Autodesk Fusion 360 part; units mm, degrees
(part 5 of 6)
ref_plane "WorkPlane4" through (0, 0, 43.2) normal (0, 0, 1) x (1, 0, 0) in component "USB — removable rear housing clamp"
sketch "USB clamp upper strap extension sketch" plane through (0, 0, 43.2) normal (0, 0, 1) x (1, 0, 0) in component "USB — removable rear housing clamp"
  line L0 (65.7, 19.7) -> (72.4, 19.7)
  line L1 (72.4, 19.7) -> (72.4, 25)
  line L2 (72.4, 25) -> (65.7, 25)
  line L3 (65.7, 25) -> (65.7, 19.7)
  dimension "d2143" = 65.7
  dimension "d2144" = 19.7
  dimension "d2145" = 6.7
  dimension "d2146" = 5.3
  constraint horizontal L0
  constraint vertical L1
  constraint horizontal L2
  constraint vertical L3
  measures "d2143" horizontal distance of origin L0.start
  measures "d2144" vertical distance of origin L0.start
  measures "d2145" horizontal distance of L0.start L0.end
  measures "d2146" vertical distance of L0.end L1.end
extrude "USB clamp upper strap extension" add sketch "USB clamp upper strap extension sketch" along normal blind 2 bodies 61 in component "USB — removable rear housing clamp"
ref_plane "WorkPlane5" through (0, 0, 35) normal (0, 0, 1) x (1, 0, 0) in component "USB — removable rear housing clamp"
sketch "USB clamp upper inward-stop stalk sketch" plane through (0, 0, 35) normal (0, 0, 1) x (1, 0, 0) in component "USB — removable rear housing clamp"
  line L0 (68.4, 23) -> (70.4, 23)
  line L1 (70.4, 23) -> (70.4, 25)
  line L2 (70.4, 25) -> (68.4, 25)
  line L3 (68.4, 25) -> (68.4, 23)
  dimension "d2151" = 68.4
  dimension "d2152" = 23
  dimension "d2153" = 2
  dimension "d2154" = 2
  constraint horizontal L0
  constraint vertical L1
  constraint horizontal L2
  constraint vertical L3
  measures "d2151" horizontal distance of origin L0.start
  measures "d2152" vertical distance of origin L0.start
  measures "d2153" horizontal distance of L0.start L0.end
  measures "d2154" vertical distance of L0.end L1.end
extrude "USB clamp upper inward-stop stalk" add sketch "USB clamp upper inward-stop stalk sketch" along normal blind 8.3 bodies 61 in component "USB — removable rear housing clamp"
ref_plane "WorkPlane6" through (0, 0, 34.9) normal (0, 0, 1) x (1, 0, 0) in component "USB — removable rear housing clamp"
sketch "Clear lower rear-cover boss from USB clamp sketch" plane through (0, 0, 34.9) normal (0, 0, 1) x (1, 0, 0) in component "USB — removable rear housing clamp"
  line L0 (65.6, 8.4) -> (72.5, 8.4)
  line L1 (72.5, 8.4) -> (72.5, 12)
  line L2 (72.5, 12) -> (65.6, 12)
  line L3 (65.6, 12) -> (65.6, 8.4)
  dimension "d2159" = 65.6
  dimension "d2160" = 8.4
  dimension "d2161" = 6.9
  dimension "d2162" = 3.6
  constraint horizontal L0
  constraint vertical L1
  constraint horizontal L2
  constraint vertical L3
  measures "d2159" horizontal distance of origin L0.start
  measures "d2160" vertical distance of origin L0.start
  measures "d2161" horizontal distance of L0.start L0.end
  measures "d2162" vertical distance of L0.end L1.end
extrude "Clear lower rear-cover boss from USB clamp" cut sketch "Clear lower rear-cover boss from USB clamp sketch" along normal blind 10.4 bodies 61 in component "USB — removable rear housing clamp"
ref_plane "WorkPlane1" through (0, 0, 21.25) normal (0, 0, 1) x (1, 0, 0)
sketch "USB parametric mounting point 2" plane through (0, 0, 21.25) normal (0, 0, 1) x (1, 0, 0)
  circle A0 centre (74.9, 8.25) radius 0.1
  dimension "d2175" = 74.9
  dimension "d2176" = 8.25
  dimension "d2177" = 0.1
  measures "d2175" horizontal distance of origin A0.centre
  measures "d2176" vertical distance of origin A0.centre
  measures "d2177" radius of A0
sketch "Negative Z orientation datum 2" plane through (0, 0, 0) normal (0, 1, 0) x (1, 0, 0)
  line L0 (0, 0) -> (0, 10)
ref_plane "WorkPlane2" through (0, 0, 30.95) normal (0, 0, 1) x (1, 0, 0)
sketch "USB parametric mounting point 6" plane through (0, 0, 30.95) normal (0, 0, 1) x (1, 0, 0)
  circle A0 centre (74.9, 23.75) radius 0.1
  dimension "d2212" = 74.9
  dimension "d2213" = 23.75
  dimension "d2214" = 0.1
  measures "d2212" horizontal distance of origin A0.centre
  measures "d2213" vertical distance of origin A0.centre
  measures "d2214" radius of A0
sketch "Negative Z orientation datum 6" plane through (0, 0, 0) normal (0, 1, 0) x (1, 0, 0)
  line L0 (0, 0) -> (0, 10)
ref_plane "WorkPlane3" through (0, 0, 21.25) normal (0, 0, 1) x (1, 0, 0)
sketch "USB parametric mounting point 7" plane through (0, 0, 21.25) normal (0, 0, 1) x (1, 0, 0)
  circle A0 centre (72.6, 8.25) radius 0.1
  dimension "d2225" = 72.6
  dimension "d2226" = 8.25
  dimension "d2227" = 0.1
  measures "d2225" horizontal distance of origin A0.centre
  measures "d2226" vertical distance of origin A0.centre
  measures "d2227" radius of A0
sketch "Negative Z orientation datum 7" plane through (0, 0, 0) normal (0, 1, 0) x (1, 0, 0)
  line L0 (0, 0) -> (0, 10)
ref_plane "WorkPlane4" through (0, 0, 30.95) normal (0, 0, 1) x (1, 0, 0)
sketch "USB parametric mounting point 8" plane through (0, 0, 30.95) normal (0, 0, 1) x (1, 0, 0)
  circle A0 centre (72.6, 23.75) radius 0.1
  dimension "d2238" = 72.6
  dimension "d2239" = 23.75
  dimension "d2240" = 0.1
  measures "d2238" horizontal distance of origin A0.centre
  measures "d2239" vertical distance of origin A0.centre
  measures "d2240" radius of A0
sketch "Negative Z orientation datum 8" plane through (0, 0, 0) normal (0, 1, 0) x (1, 0, 0)
  line L0 (0, 0) -> (0, 10)
ref_plane "WorkPlane1" through (0, 0, 16.5) normal (0, 0, 1) x (1, 0, 0) in component "Chamber / sealed L cartridge concept"
sketch "L sampling cartridge sketch" plane through (0, 0, 16.5) normal (0, 0, 1) x (1, 0, 0) in component "Chamber / sealed L cartridge concept"
  line L0 (2.9, 87) -> (72.1, 87)
  line L1 (72.1, 87) -> (72.1, 122.1)
  line L2 (72.1, 122.1) -> (2.9, 122.1)
  line L3 (2.9, 122.1) -> (2.9, 87)
  dimension "d2267" = 2.9
  dimension "d2268" = 87
  constraint horizontal L0
  constraint vertical L1
  constraint horizontal L2
  constraint vertical L3
  measures "d2267" horizontal distance of origin L0.start
  measures "d2268" vertical distance of origin L0.start
extrude "L sampling cartridge" add sketch "L sampling cartridge sketch" along normal blind 32.3 separate body makes body 85 in component "Chamber / sealed L cartridge concept"
ref_plane "WorkPlane2" through (0, 0, 16.5) normal (0, 0, 1) x (1, 0, 0) in component "Chamber / sealed L cartridge concept"
sketch "L sampling cartridge side column sketch" plane through (0, 0, 16.5) normal (0, 0, 1) x (1, 0, 0) in component "Chamber / sealed L cartridge concept"
  line L0 (45.6, 30) -> (72.1, 30)
  line L1 (72.1, 30) -> (72.1, 122.1)
  line L2 (72.1, 122.1) -> (45.6, 122.1)
  line L3 (45.6, 122.1) -> (45.6, 30)
  dimension "d2275" = 45.6
  dimension "d2276" = 30
  constraint horizontal L0
  constraint vertical L1
  constraint horizontal L2
  constraint vertical L3
  measures "d2275" horizontal distance of origin L0.start
  measures "d2276" vertical distance of origin L0.start
extrude "L sampling cartridge side column" add sketch "L sampling cartridge side column sketch" along normal blind 32.3 bodies 85 in component "Chamber / sealed L cartridge concept"
ref_plane "WorkPlane3" through (0, 0, 18.5) normal (0, 0, 1) x (1, 0, 0) in component "Chamber / sealed L cartridge concept"
sketch "Direct upper gas cavity sketch" plane through (0, 0, 18.5) normal (0, 0, 1) x (1, 0, 0) in component "Chamber / sealed L cartridge concept"
  line L0 (4.9, 89) -> (70.1, 89)
  line L1 (70.1, 89) -> (70.1, 120.1)
  line L2 (70.1, 120.1) -> (4.9, 120.1)
  line L3 (4.9, 120.1) -> (4.9, 89)
  dimension "d2283" = 4.9
  dimension "d2284" = 89
  dimension "d2285" = 65.2
  dimension "d2286" = 31.1
  constraint horizontal L0
  constraint vertical L1
  constraint horizontal L2
  constraint vertical L3
  measures "d2283" horizontal distance of origin L0.start
  measures "d2284" vertical distance of origin L0.start
  measures "d2285" horizontal distance of L0.start L0.end
  measures "d2286" vertical distance of L0.end L1.end
extrude "Direct upper gas cavity" cut sketch "Direct upper gas cavity sketch" along normal blind 56 bodies 85 in component "Chamber / sealed L cartridge concept"
ref_plane "WorkPlane4" through (0, 0, 18.5) normal (0, 0, 1) x (1, 0, 0) in component "Chamber / sealed L cartridge concept"
sketch "Direct connected side gas cavity sketch" plane through (0, 0, 18.5) normal (0, 0, 1) x (1, 0, 0) in component "Chamber / sealed L cartridge concept"
  line L0 (47.6, 32) -> (70.1, 32)
  line L1 (70.1, 32) -> (70.1, 120.1)
  line L2 (70.1, 120.1) -> (47.6, 120.1)
  line L3 (47.6, 120.1) -> (47.6, 32)
  dimension "d2291" = 47.6
  dimension "d2292" = 32
  dimension "d2293" = 22.5
  dimension "d2294" = 88.1
  constraint horizontal L0
  constraint vertical L1
  constraint horizontal L2
  constraint vertical L3
  measures "d2291" horizontal distance of origin L0.start
  measures "d2292" vertical distance of origin L0.start
  measures "d2293" horizontal distance of L0.start L0.end
  measures "d2294" vertical distance of L0.end L1.end
extrude "Direct connected side gas cavity" cut sketch "Direct connected side gas cavity sketch" along normal blind 56 bodies 85 in component "Chamber / sealed L cartridge concept"
ref_plane "WorkPlane5" through (0, 0, 16.5) normal (0, 0, 1) x (1, 0, 0) in component "Chamber / sealed L cartridge concept"
sketch "Joined M3 exclusion wall stock sketch" plane through (0, 0, 16.5) normal (0, 0, 1) x (1, 0, 0) in component "Chamber / sealed L cartridge concept"
  circle A0 centre (6, 119) radius 6.5
  dimension "d2299" = 6
  dimension "d2300" = 119
  dimension "d2301" = 6.5
  measures "d2299" horizontal distance of origin A0.centre
  measures "d2300" vertical distance of origin A0.centre
  measures "d2301" radius of A0
extrude "Joined M3 exclusion wall stock" add sketch "Joined M3 exclusion wall stock sketch" along normal blind 32.3 bodies 85 in component "Chamber / sealed L cartridge concept"
ref_plane "WorkPlane6" through (0, 0, 16.5) normal (0, 0, 1) x (1, 0, 0) in component "Chamber / sealed L cartridge concept"
sketch "Joined M3 exclusion wall stock sketch (1)" plane through (0, 0, 16.5) normal (0, 0, 1) x (1, 0, 0) in component "Chamber / sealed L cartridge concept"
  circle A0 centre (69, 119) radius 6.5
  dimension "d2306" = 69
  dimension "d2307" = 119
  dimension "d2308" = 6.5
  measures "d2306" horizontal distance of origin A0.centre
  measures "d2307" vertical distance of origin A0.centre
  measures "d2308" radius of A0
extrude "Joined M3 exclusion wall stock (1)" add sketch "Joined M3 exclusion wall stock sketch (1)" along normal blind 32.3 bodies 85 in component "Chamber / sealed L cartridge concept"
ref_plane "WorkPlane7" through (0, 0, 16.5) normal (0, 0, 1) x (1, 0, 0) in component "Chamber / sealed L cartridge concept"
sketch "Joined 2 mm retainer notch wall stock sketch" plane through (0, 0, 16.5) normal (0, 0, 1) x (1, 0, 0) in component "Chamber / sealed L cartridge concept"
  line L0 (2.9, 112.8) -> (20.1, 112.8)
  line L1 (20.1, 112.8) -> (20.1, 122.1)
  line L2 (20.1, 122.1) -> (2.9, 122.1)
  line L3 (2.9, 122.1) -> (2.9, 112.8)
  dimension "d2313" = 2.9
  dimension "d2314" = 112.8
  dimension "d2315" = 17.2
  dimension "d2316" = 9.3
  constraint horizontal L0
  constraint vertical L1
  constraint horizontal L2
  constraint vertical L3
  measures "d2313" horizontal distance of origin L0.start
  measures "d2314" vertical distance of origin L0.start
  measures "d2315" horizontal distance of L0.start L0.end
  measures "d2316" vertical distance of L0.end L1.end
extrude "Joined 2 mm retainer notch wall stock" add sketch "Joined 2 mm retainer notch wall stock sketch" along normal blind 32.3 bodies 85 in component "Chamber / sealed L cartridge concept"
ref_plane "WorkPlane8" through (0, 0, 16.5) normal (0, 0, 1) x (1, 0, 0) in component "Chamber / sealed L cartridge concept"
sketch "Joined isolated housing post tunnel sketch" plane through (0, 0, 16.5) normal (0, 0, 1) x (1, 0, 0) in component "Chamber / sealed L cartridge concept"
  circle A0 centre (8.8, 94.7) radius 5.8
  dimension "d2321" = 8.8
  dimension "d2322" = 94.7
  dimension "d2323" = 5.8
  measures "d2321" horizontal distance of origin A0.centre
  measures "d2322" vertical distance of origin A0.centre
  measures "d2323" radius of A0
extrude "Joined isolated housing post tunnel" add sketch "Joined isolated housing post tunnel sketch" along normal blind 32.3 bodies 85 in component "Chamber / sealed L cartridge concept"
ref_plane "WorkPlane9" through (0, 0, 16.5) normal (0, 0, 1) x (1, 0, 0) in component "Chamber / sealed L cartridge concept"
sketch "Joined isolated housing post tunnel sketch (1)" plane through (0, 0, 16.5) normal (0, 0, 1) x (1, 0, 0) in component "Chamber / sealed L cartridge concept"
  circle A0 centre (59.2, 115.4) radius 5.8
  dimension "d2328" = 59.2
  dimension "d2329" = 115.4
  dimension "d2330" = 5.8
  measures "d2328" horizontal distance of origin A0.centre
  measures "d2329" vertical distance of origin A0.centre
  measures "d2330" radius of A0
extrude "Joined isolated housing post tunnel (1)" add sketch "Joined isolated housing post tunnel sketch (1)" along normal blind 32.3 bodies 85 in component "Chamber / sealed L cartridge concept"
ref_plane "WorkPlane10" through (0, 0, 15.5) normal (0, 0, 1) x (1, 0, 0) in component "Chamber / sealed L cartridge concept"
sketch "Trim stock outside left outline sketch" plane through (0, 0, 15.5) normal (0, 0, 1) x (1, 0, 0) in component "Chamber / sealed L cartridge concept"
  line L0 (-7.1, -10) -> (2.9, -10)
  line L1 (2.9, -10) -> (2.9, 135)
  line L2 (2.9, 135) -> (-7.1, 135)
  line L3 (-7.1, 135) -> (-7.1, -10)
  dimension "d2335" = 7.1
  dimension "d2336" = 10
  dimension "d2337" = 10
  dimension "d2338" = 145
  constraint horizontal L0
  constraint vertical L1
  constraint horizontal L2
  constraint vertical L3
  measures "d2335" horizontal distance of origin L0.start
  measures "d2336" vertical distance of origin L0.start
  measures "d2337" horizontal distance of L0.start L0.end
  measures "d2338" vertical distance of L0.end L1.end
extrude "Trim stock outside left outline" cut sketch "Trim stock outside left outline sketch" along normal blind 112 bodies 85 in component "Chamber / sealed L cartridge concept"
ref_plane "WorkPlane11" through (0, 0, 15.5) normal (0, 0, 1) x (1, 0, 0) in component "Chamber / sealed L cartridge concept"
sketch "Trim stock outside right outline sketch" plane through (0, 0, 15.5) normal (0, 0, 1) x (1, 0, 0) in component "Chamber / sealed L cartridge concept"
  line L0 (72.1, -10) -> (82.1, -10)
  line L1 (82.1, -10) -> (82.1, 135)
  line L2 (82.1, 135) -> (72.1, 135)
  line L3 (72.1, 135) -> (72.1, -10)
  dimension "d2343" = 72.1
  dimension "d2344" = 10
  dimension "d2345" = 10
  dimension "d2346" = 145
  constraint horizontal L0
  constraint vertical L1
  constraint horizontal L2
  constraint vertical L3
  measures "d2343" horizontal distance of origin L0.start
  measures "d2344" vertical distance of origin L0.start
  measures "d2345" horizontal distance of L0.start L0.end
  measures "d2346" vertical distance of L0.end L1.end
extrude "Trim stock outside right outline" cut sketch "Trim stock outside right outline sketch" along normal blind 112 bodies 85 in component "Chamber / sealed L cartridge concept"
ref_plane "WorkPlane12" through (0, 0, 15.5) normal (0, 0, 1) x (1, 0, 0) in component "Chamber / sealed L cartridge concept"
sketch "Trim stock outside upper outline sketch" plane through (0, 0, 15.5) normal (0, 0, 1) x (1, 0, 0) in component "Chamber / sealed L cartridge concept"
  line L0 (-7.1, 122.1) -> (82.1, 122.1)
  line L1 (82.1, 122.1) -> (82.1, 132.1)
  line L2 (82.1, 132.1) -> (-7.1, 132.1)
  line L3 (-7.1, 132.1) -> (-7.1, 122.1)
  dimension "d2351" = 7.1
  dimension "d2352" = 122.1
  dimension "d2353" = 89.2
  dimension "d2354" = 10
  constraint horizontal L0
  constraint vertical L1
  constraint horizontal L2
  constraint vertical L3
  measures "d2351" horizontal distance of origin L0.start
  measures "d2352" vertical distance of origin L0.start
  measures "d2353" horizontal distance of L0.start L0.end
  measures "d2354" vertical distance of L0.end L1.end
extrude "Trim stock outside upper outline" cut sketch "Trim stock outside upper outline sketch" along normal blind 112 bodies 85 in component "Chamber / sealed L cartridge concept"
fillet "Housing clearance top corner rounds" radius 3.1 2 edges at (2.9, 122.1, 32.65) (72.1, 122.1, 32.65) on bodies 85 in component "Chamber / sealed L cartridge concept"
ref_plane "WorkPlane13" through (0, 0, 15.5) normal (0, 0, 1) x (1, 0, 0) in component "Chamber / sealed L cartridge concept"
sketch "Cartridge upper M3 post clearance sketch" plane through (0, 0, 15.5) normal (0, 0, 1) x (1, 0, 0) in component "Chamber / sealed L cartridge concept"
  circle A0 centre (6, 119) radius 4.5
  dimension "d2361" = 6
  dimension "d2362" = 119
  dimension "d2363" = 4.5
  measures "d2361" horizontal distance of origin A0.centre
  measures "d2362" vertical distance of origin A0.centre
  measures "d2363" radius of A0
extrude "Cartridge upper M3 post clearance" cut sketch "Cartridge upper M3 post clearance sketch" along normal blind 112 bodies 85 in component "Chamber / sealed L cartridge concept"
ref_plane "WorkPlane14" through (0, 0, 15.5) normal (0, 0, 1) x (1, 0, 0) in component "Chamber / sealed L cartridge concept"
sketch "Cartridge upper M3 post clearance sketch (1)" plane through (0, 0, 15.5) normal (0, 0, 1) x (1, 0, 0) in component "Chamber / sealed L cartridge concept"
  circle A0 centre (69, 119) radius 4.5
  dimension "d2368" = 69
  dimension "d2369" = 119
  dimension "d2370" = 4.5
  measures "d2368" horizontal distance of origin A0.centre
  measures "d2369" vertical distance of origin A0.centre
  measures "d2370" radius of A0
extrude "Cartridge upper M3 post clearance (1)" cut sketch "Cartridge upper M3 post clearance sketch (1)" along normal blind 112 bodies 85 in component "Chamber / sealed L cartridge concept"
ref_plane "WorkPlane15" through (0, 0, 15.5) normal (0, 0, 1) x (1, 0, 0) in component "Chamber / sealed L cartridge concept"
sketch "Cartridge upper display retainer service notch sketch" plane through (0, 0, 15.5) normal (0, 0, 1) x (1, 0, 0) in component "Chamber / sealed L cartridge concept"
  line L0 (1.9, 114.8) -> (18.1, 114.8)
  line L1 (18.1, 114.8) -> (18.1, 125)
  line L2 (18.1, 125) -> (1.9, 125)
  line L3 (1.9, 125) -> (1.9, 114.8)
  dimension "d2375" = 1.9
  dimension "d2376" = 114.8
  dimension "d2377" = 16.2
  dimension "d2378" = 10.2
  constraint horizontal L0
  constraint vertical L1
  constraint horizontal L2
  constraint vertical L3
  measures "d2375" horizontal distance of origin L0.start
  measures "d2376" vertical distance of origin L0.start
  measures "d2377" horizontal distance of L0.start L0.end
  measures "d2378" vertical distance of L0.end L1.end
extrude "Cartridge upper display retainer service notch" cut sketch "Cartridge upper display retainer service notch sketch" along normal blind 112 bodies 85 in component "Chamber / sealed L cartridge concept"
ref_plane "WorkPlane16" through (0, 0, 16.4) normal (0, 0, 1) x (1, 0, 0) in component "Chamber / sealed L cartridge concept"
sketch "Stationary post withdrawal passage sketch" plane through (0, 0, 16.4) normal (0, 0, 1) x (1, 0, 0) in component "Chamber / sealed L cartridge concept"
  circle A0 centre (8.8, 94.7) radius 3.8
  dimension "d2383" = 8.8
  dimension "d2384" = 94.7
  dimension "d2385" = 3.8
  measures "d2383" horizontal distance of origin A0.centre
  measures "d2384" vertical distance of origin A0.centre
  measures "d2385" radius of A0
extrude "Stationary post withdrawal passage" cut sketch "Stationary post withdrawal passage sketch" along normal blind 30.4 bodies 85 in component "Chamber / sealed L cartridge concept"
ref_plane "WorkPlane17" through (0, 0, 46.7) normal (0, 0, 1) x (1, 0, 0) in component "Chamber / sealed L cartridge concept"
sketch "M2 mounting roof clearance sketch" plane through (0, 0, 46.7) normal (0, 0, 1) x (1, 0, 0) in component "Chamber / sealed L cartridge concept"
  circle A0 centre (8.8, 94.7) radius 1.2
  dimension "d2390" = 8.8
  dimension "d2391" = 94.7
  dimension "d2392" = 1.2
  measures "d2390" horizontal distance of origin A0.centre
  measures "d2391" vertical distance of origin A0.centre
  measures "d2392" radius of A0
extrude "M2 mounting roof clearance" cut sketch "M2 mounting roof clearance sketch" along normal blind 2.2 bodies 85 in component "Chamber / sealed L cartridge concept"
ref_plane "WorkPlane18" through (0, 0, 16.4) normal (0, 0, 1) x (1, 0, 0) in component "Chamber / sealed L cartridge concept"
sketch "Stationary post withdrawal passage sketch (1)" plane through (0, 0, 16.4) normal (0, 0, 1) x (1, 0, 0) in component "Chamber / sealed L cartridge concept"
  circle A0 centre (59.2, 115.4) radius 3.8
  dimension "d2397" = 59.2
  dimension "d2398" = 115.4
  dimension "d2399" = 3.8
  measures "d2397" horizontal distance of origin A0.centre
  measures "d2398" vertical distance of origin A0.centre
  measures "d2399" radius of A0
extrude "Stationary post withdrawal passage (1)" cut sketch "Stationary post withdrawal passage sketch (1)" along normal blind 30.4 bodies 85 in component "Chamber / sealed L cartridge concept"
ref_plane "WorkPlane19" through (0, 0, 46.7) normal (0, 0, 1) x (1, 0, 0) in component "Chamber / sealed L cartridge concept"
sketch "M2 mounting roof clearance sketch (1)" plane through (0, 0, 46.7) normal (0, 0, 1) x (1, 0, 0) in component "Chamber / sealed L cartridge concept"
  circle A0 centre (59.2, 115.4) radius 1.2
  dimension "d2404" = 59.2
  dimension "d2405" = 115.4
  dimension "d2406" = 1.2
  measures "d2404" horizontal distance of origin A0.centre
  measures "d2405" vertical distance of origin A0.centre
  measures "d2406" radius of A0
extrude "M2 mounting roof clearance (1)" cut sketch "M2 mounting roof clearance sketch (1)" along normal blind 2.2 bodies 85 in component "Chamber / sealed L cartridge concept"
ref_plane "WorkPlane20" through (0, 0, 42.8) normal (0, 0, 1) x (1, 0, 0) in component "Chamber / sealed L cartridge concept"
sketch "Lid boss wall support sketch" plane through (0, 0, 42.8) normal (0, 0, 1) x (1, 0, 0) in component "Chamber / sealed L cartridge concept"
  line L0 (13.75, 87) -> (21.05, 87)
  line L1 (21.05, 87) -> (21.05, 92.6)
  line L2 (21.05, 92.6) -> (13.75, 92.6)
  line L3 (13.75, 92.6) -> (13.75, 87)
  dimension "d2411" = 13.75
  dimension "d2412" = 87
  dimension "d2413" = 7.3
  dimension "d2414" = 5.6
  constraint horizontal L0
  constraint vertical L1
  constraint horizontal L2
  constraint vertical L3
  measures "d2411" horizontal distance of origin L0.start
  measures "d2412" vertical distance of origin L0.start
  measures "d2413" horizontal distance of L0.start L0.end
  measures "d2414" vertical distance of L0.end L1.end
extrude "Lid boss wall support" add sketch "Lid boss wall support sketch" along normal blind 6 bodies 85 in component "Chamber / sealed L cartridge concept"
ref_plane "WorkPlane21" through (0, 0, 42.8) normal (0, 0, 1) x (1, 0, 0) in component "Chamber / sealed L cartridge concept"
sketch "M2 lid boss with 2 mm radial plastic sketch" plane through (0, 0, 42.8) normal (0, 0, 1) x (1, 0, 0) in component "Chamber / sealed L cartridge concept"
  circle A0 centre (17.4, 92.6) radius 3.65
  dimension "d2419" = 17.4
  dimension "d2420" = 92.6
  dimension "d2421" = 3.65
  measures "d2419" horizontal distance of origin A0.centre
  measures "d2420" vertical distance of origin A0.centre
  measures "d2421" radius of A0
extrude "M2 lid boss with 2 mm radial plastic" add sketch "M2 lid boss with 2 mm radial plastic sketch" along normal blind 6 bodies 85 in component "Chamber / sealed L cartridge concept"
ref_plane "WorkPlane22" through (0, 0, 44.8) normal (0, 0, 1) x (1, 0, 0) in component "Chamber / sealed L cartridge concept"
sketch "Sketch22" plane through (0, 0, 44.8) normal (0, 0, 1) x (1, 0, 0) in component "Chamber / sealed L cartridge concept"
  circle A0 centre (17.4, 92.6) radius 1.65
  dimension "d2426" = 17.4
  dimension "d2427" = 92.6
  dimension "d2428" = 1.65
  measures "d2426" horizontal distance of origin A0.centre
  measures "d2427" vertical distance of origin A0.centre
  measures "d2428" radius of A0
extrude "M2 lid insert pocket — supplier fit pending" cut sketch "Sketch22" along normal blind 4.1 bodies 85 in component "Chamber / sealed L cartridge concept"
ref_plane "WorkPlane23" through (0, 0, 42.8) normal (0, 0, 1) x (1, 0, 0) in component "Chamber / sealed L cartridge concept"
sketch "Lid boss wall support sketch (1)" plane through (0, 0, 42.8) normal (0, 0, 1) x (1, 0, 0) in component "Chamber / sealed L cartridge concept"
  line L0 (2.9, 106.95) -> (12.9, 106.95)
  line L1 (12.9, 106.95) -> (12.9, 114.25)
  line L2 (12.9, 114.25) -> (2.9, 114.25)
  line L3 (2.9, 114.25) -> (2.9, 106.95)
  dimension "d2433" = 2.9
  dimension "d2434" = 106.95
  dimension "d2435" = 10
  dimension "d2436" = 7.3
  constraint horizontal L0
  constraint vertical L1
  constraint horizontal L2
  constraint vertical L3
  measures "d2433" horizontal distance of origin L0.start
  measures "d2434" vertical distance of origin L0.start
  measures "d2435" horizontal distance of L0.start L0.end
  measures "d2436" vertical distance of L0.end L1.end
extrude "Lid boss wall support (1)" add sketch "Lid boss wall support sketch (1)" along normal blind 6 bodies 85 in component "Chamber / sealed L cartridge concept"
ref_plane "WorkPlane24" through (0, 0, 42.8) normal (0, 0, 1) x (1, 0, 0) in component "Chamber / sealed L cartridge concept"
sketch "M2 lid boss with 2 mm radial plastic sketch (1)" plane through (0, 0, 42.8) normal (0, 0, 1) x (1, 0, 0) in component "Chamber / sealed L cartridge concept"
  circle A0 centre (12.9, 110.6) radius 3.65
  dimension "d2441" = 12.9
  dimension "d2442" = 110.6
  dimension "d2443" = 3.65
  measures "d2441" horizontal distance of origin A0.centre
  measures "d2442" vertical distance of origin A0.centre
  measures "d2443" radius of A0
extrude "M2 lid boss with 2 mm radial plastic (1)" add sketch "M2 lid boss with 2 mm radial plastic sketch (1)" along normal blind 6 bodies 85 in component "Chamber / sealed L cartridge concept"
ref_plane "WorkPlane25" through (0, 0, 44.8) normal (0, 0, 1) x (1, 0, 0) in component "Chamber / sealed L cartridge concept"
sketch "Sketch25" plane through (0, 0, 44.8) normal (0, 0, 1) x (1, 0, 0) in component "Chamber / sealed L cartridge concept"
  circle A0 centre (12.9, 110.6) radius 1.65
  dimension "d2448" = 12.9
  dimension "d2449" = 110.6
  dimension "d2450" = 1.65
  measures "d2448" horizontal distance of origin A0.centre
  measures "d2449" vertical distance of origin A0.centre
  measures "d2450" radius of A0
extrude "M2 lid insert pocket — supplier fit pending (1)" cut sketch "Sketch25" along normal blind 4.1 bodies 85 in component "Chamber / sealed L cartridge concept"
ref_plane "WorkPlane26" through (0, 0, 42.8) normal (0, 0, 1) x (1, 0, 0) in component "Chamber / sealed L cartridge concept"
sketch "Lid boss wall support sketch (2)" plane through (0, 0, 42.8) normal (0, 0, 1) x (1, 0, 0) in component "Chamber / sealed L cartridge concept"
  line L0 (66.5, 79.85) -> (72.1, 79.85)
  line L1 (72.1, 79.85) -> (72.1, 87.15)
  line L2 (72.1, 87.15) -> (66.5, 87.15)
  line L3 (66.5, 87.15) -> (66.5, 79.85)
  dimension "d2455" = 66.5
  dimension "d2456" = 79.85
  dimension "d2457" = 5.6
  dimension "d2458" = 7.3
  constraint horizontal L0
  constraint vertical L1
  constraint horizontal L2
  constraint vertical L3
  measures "d2455" horizontal distance of origin L0.start
  measures "d2456" vertical distance of origin L0.start
  measures "d2457" horizontal distance of L0.start L0.end
  measures "d2458" vertical distance of L0.end L1.end
extrude "Lid boss wall support (2)" add sketch "Lid boss wall support sketch (2)" along normal blind 6 bodies 85 in component "Chamber / sealed L cartridge concept"
ref_plane "WorkPlane27" through (0, 0, 42.8) normal (0, 0, 1) x (1, 0, 0) in component "Chamber / sealed L cartridge concept"
sketch "M2 lid boss with 2 mm radial plastic sketch (2)" plane through (0, 0, 42.8) normal (0, 0, 1) x (1, 0, 0) in component "Chamber / sealed L cartridge concept"
  circle A0 centre (66.5, 83.5) radius 3.65
  dimension "d2463" = 66.5
  dimension "d2464" = 83.5
  dimension "d2465" = 3.65
  measures "d2463" horizontal distance of origin A0.centre
  measures "d2464" vertical distance of origin A0.centre
  measures "d2465" radius of A0
extrude "M2 lid boss with 2 mm radial plastic (2)" add sketch "M2 lid boss with 2 mm radial plastic sketch (2)" along normal blind 6 bodies 85 in component "Chamber / sealed L cartridge concept"
ref_plane "WorkPlane28" through (0, 0, 44.8) normal (0, 0, 1) x (1, 0, 0) in component "Chamber / sealed L cartridge concept"
sketch "Sketch28" plane through (0, 0, 44.8) normal (0, 0, 1) x (1, 0, 0) in component "Chamber / sealed L cartridge concept"
  circle A0 centre (66.5, 83.5) radius 1.65
  dimension "d2470" = 66.5
  dimension "d2471" = 83.5
  dimension "d2472" = 1.65
  measures "d2470" horizontal distance of origin A0.centre
  measures "d2471" vertical distance of origin A0.centre
  measures "d2472" radius of A0
extrude "M2 lid insert pocket — supplier fit pending (2)" cut sketch "Sketch28" along normal blind 4.1 bodies 85 in component "Chamber / sealed L cartridge concept"
ref_plane "WorkPlane29" through (0, 0, 42.8) normal (0, 0, 1) x (1, 0, 0) in component "Chamber / sealed L cartridge concept"
sketch "Lid boss wall support sketch (3)" plane through (0, 0, 42.8) normal (0, 0, 1) x (1, 0, 0) in component "Chamber / sealed L cartridge concept"
  line L0 (66.5, 106.85) -> (72.1, 106.85)
  line L1 (72.1, 106.85) -> (72.1, 114.15)
  line L2 (72.1, 114.15) -> (66.5, 114.15)
  line L3 (66.5, 114.15) -> (66.5, 106.85)
  dimension "d2477" = 66.5
  dimension "d2478" = 106.85
  dimension "d2479" = 5.6
  dimension "d2480" = 7.3
  constraint horizontal L0
  constraint vertical L1
  constraint horizontal L2
  constraint vertical L3
  measures "d2477" horizontal distance of origin L0.start
  measures "d2478" vertical distance of origin L0.start
  measures "d2479" horizontal distance of L0.start L0.end
  measures "d2480" vertical distance of L0.end L1.end
extrude "Lid boss wall support (3)" add sketch "Lid boss wall support sketch (3)" along normal blind 6 bodies 85 in component "Chamber / sealed L cartridge concept"
ref_plane "WorkPlane30" through (0, 0, 42.8) normal (0, 0, 1) x (1, 0, 0) in component "Chamber / sealed L cartridge concept"
sketch "M2 lid boss with 2 mm radial plastic sketch (3)" plane through (0, 0, 42.8) normal (0, 0, 1) x (1, 0, 0) in component "Chamber / sealed L cartridge concept"
  circle A0 centre (66.5, 110.5) radius 3.65
  dimension "d2485" = 66.5
  dimension "d2486" = 110.5
  dimension "d2487" = 3.65
  measures "d2485" horizontal distance of origin A0.centre
  measures "d2486" vertical distance of origin A0.centre
  measures "d2487" radius of A0
extrude "M2 lid boss with 2 mm radial plastic (3)" add sketch "M2 lid boss with 2 mm radial plastic sketch (3)" along normal blind 6 bodies 85 in component "Chamber / sealed L cartridge concept"
ref_plane "WorkPlane31" through (0, 0, 44.8) normal (0, 0, 1) x (1, 0, 0) in component "Chamber / sealed L cartridge concept"
sketch "Sketch31" plane through (0, 0, 44.8) normal (0, 0, 1) x (1, 0, 0) in component "Chamber / sealed L cartridge concept"
  circle A0 centre (66.5, 110.5) radius 1.65
  dimension "d2492" = 66.5
  dimension "d2493" = 110.5
  dimension "d2494" = 1.65
  measures "d2492" horizontal distance of origin A0.centre
  measures "d2493" vertical distance of origin A0.centre
  measures "d2494" radius of A0
extrude "M2 lid insert pocket — supplier fit pending (3)" cut sketch "Sketch31" along normal blind 4.1 bodies 85 in component "Chamber / sealed L cartridge concept"
ref_plane "WorkPlane32" through (0, 0, 42.8) normal (0, 0, 1) x (1, 0, 0) in component "Chamber / sealed L cartridge concept"
sketch "Lid boss wall support sketch (4)" plane through (0, 0, 42.8) normal (0, 0, 1) x (1, 0, 0) in component "Chamber / sealed L cartridge concept"
  line L0 (45.6, 30.35) -> (51.2, 30.35)
  line L1 (51.2, 30.35) -> (51.2, 37.65)
  line L2 (51.2, 37.65) -> (45.6, 37.65)
  line L3 (45.6, 37.65) -> (45.6, 30.35)
  dimension "d2499" = 45.6
  dimension "d2500" = 30.35
  dimension "d2501" = 5.6
  dimension "d2502" = 7.3
  constraint horizontal L0
  constraint vertical L1
  constraint horizontal L2
  constraint vertical L3
  measures "d2499" horizontal distance of origin L0.start
  measures "d2500" vertical distance of origin L0.start
  measures "d2501" horizontal distance of L0.start L0.end
  measures "d2502" vertical distance of L0.end L1.end
extrude "Lid boss wall support (4)" add sketch "Lid boss wall support sketch (4)" along normal blind 6 bodies 85 in component "Chamber / sealed L cartridge concept"
ref_plane "WorkPlane33" through (0, 0, 42.8) normal (0, 0, 1) x (1, 0, 0) in component "Chamber / sealed L cartridge concept"
sketch "M2 lid boss with 2 mm radial plastic sketch (4)" plane through (0, 0, 42.8) normal (0, 0, 1) x (1, 0, 0) in component "Chamber / sealed L cartridge concept"
  circle A0 centre (51.2, 34) radius 3.65
  dimension "d2507" = 51.2
  dimension "d2508" = 34
  dimension "d2509" = 3.65
  measures "d2507" horizontal distance of origin A0.centre
  measures "d2508" vertical distance of origin A0.centre
  measures "d2509" radius of A0
extrude "M2 lid boss with 2 mm radial plastic (4)" add sketch "M2 lid boss with 2 mm radial plastic sketch (4)" along normal blind 6 bodies 85 in component "Chamber / sealed L cartridge concept"
ref_plane "WorkPlane34" through (0, 0, 44.8) normal (0, 0, 1) x (1, 0, 0) in component "Chamber / sealed L cartridge concept"
sketch "Sketch34" plane through (0, 0, 44.8) normal (0, 0, 1) x (1, 0, 0) in component "Chamber / sealed L cartridge concept"
  circle A0 centre (51.2, 34) radius 1.65
  dimension "d2514" = 51.2
  dimension "d2515" = 34
  dimension "d2516" = 1.65
  measures "d2514" horizontal distance of origin A0.centre
  measures "d2515" vertical distance of origin A0.centre
  measures "d2516" radius of A0
extrude "M2 lid insert pocket — supplier fit pending (4)" cut sketch "Sketch34" along normal blind 4.1 bodies 85 in component "Chamber / sealed L cartridge concept"
ref_plane "WorkPlane35" through (0, 0, 42.8) normal (0, 0, 1) x (1, 0, 0) in component "Chamber / sealed L cartridge concept"
sketch "Lid boss wall support sketch (5)" plane through (0, 0, 42.8) normal (0, 0, 1) x (1, 0, 0) in component "Chamber / sealed L cartridge concept"
  line L0 (66.5, 30.35) -> (72.1, 30.35)
  line L1 (72.1, 30.35) -> (72.1, 37.65)
  line L2 (72.1, 37.65) -> (66.5, 37.65)
  line L3 (66.5, 37.65) -> (66.5, 30.35)
  dimension "d2521" = 66.5
  dimension "d2522" = 30.35
  dimension "d2523" = 5.6
  dimension "d2524" = 7.3
  constraint horizontal L0
  constraint vertical L1
  constraint horizontal L2
  constraint vertical L3
  measures "d2521" horizontal distance of origin L0.start
  measures "d2522" vertical distance of origin L0.start
  measures "d2523" horizontal distance of L0.start L0.end
  measures "d2524" vertical distance of L0.end L1.end
extrude "Lid boss wall support (5)" add sketch "Lid boss wall support sketch (5)" along normal blind 6 bodies 85 in component "Chamber / sealed L cartridge concept"
ref_plane "WorkPlane36" through (0, 0, 42.8) normal (0, 0, 1) x (1, 0, 0) in component "Chamber / sealed L cartridge concept"
sketch "M2 lid boss with 2 mm radial plastic sketch (5)" plane through (0, 0, 42.8) normal (0, 0, 1) x (1, 0, 0) in component "Chamber / sealed L cartridge concept"
  circle A0 centre (66.5, 34) radius 3.65
  dimension "d2529" = 66.5
  dimension "d2530" = 34
  dimension "d2531" = 3.65
  measures "d2529" horizontal distance of origin A0.centre
  measures "d2530" vertical distance of origin A0.centre
  measures "d2531" radius of A0
extrude "M2 lid boss with 2 mm radial plastic (5)" add sketch "M2 lid boss with 2 mm radial plastic sketch (5)" along normal blind 6 bodies 85 in component "Chamber / sealed L cartridge concept"
ref_plane "WorkPlane37" through (0, 0, 44.8) normal (0, 0, 1) x (1, 0, 0) in component "Chamber / sealed L cartridge concept"
sketch "Sketch37" plane through (0, 0, 44.8) normal (0, 0, 1) x (1, 0, 0) in component "Chamber / sealed L cartridge concept"
  circle A0 centre (66.5, 34) radius 1.65
  dimension "d2536" = 66.5
  dimension "d2537" = 34
  dimension "d2538" = 1.65
  measures "d2536" horizontal distance of origin A0.centre
  measures "d2537" vertical distance of origin A0.centre
  measures "d2538" radius of A0
extrude "M2 lid insert pocket — supplier fit pending (5)" cut sketch "Sketch37" along normal blind 4.1 bodies 85 in component "Chamber / sealed L cartridge concept"
ref_plane "WorkPlane38" through (-1, 0, 0) normal (1, 0, 0) x (0, 1, 0) in component "Chamber / sealed L cartridge concept"
sketch "Gas fitting chamber wall passages sketch" plane through (-1, 0, 0) normal (1, 0, 0) x (0, 0, -1) in component "Chamber / sealed L cartridge concept"
  circle A0 centre (-23, 105) radius 4.1
  dimension "d2544" = 105
  dimension "d2545" = 4.1
  measures "d2544" vertical distance of origin A0.centre
  measures "d2545" radius of A0
extrude "Gas fitting chamber wall passages" cut sketch "Gas fitting chamber wall passages sketch" along normal blind 77 bodies 85 in component "Chamber / sealed L cartridge concept"
ref_plane "WorkPlane39" through (42, 0, 0) normal (1, 0, 0) x (0, 1, 0) in component "Chamber / sealed L cartridge concept"
sketch "Sketch39" plane through (42, 0, 0) normal (1, 0, 0) x (0, 0, -1) in component "Chamber / sealed L cartridge concept"
  circle A0 centre (-44.5, 73) radius 2.4
  dimension "d2550" = 44.5
  dimension "d2551" = 73
  dimension "d2552" = 2.4
  measures "d2550" horizontal distance of origin A0.centre
  measures "d2551" vertical distance of origin A0.centre
  measures "d2552" radius of A0
extrude "Wired sensor feedthrough opening — gland fit pending" cut sketch "Sketch39" along normal blind 6 bodies 85 in component "Chamber / sealed L cartridge concept"
component "01 Tapered printed housing" placed x (1, 0, 0) y (0, 1, 0) z (0, 0, 1) at (0, 0, 0)
component "02 Single rear cover" placed x (1, 0, 0) y (0, 1, 0) z (0, 0, 1) at (0, 0, 0)
component "03 Guition factory casing — measured envelope" placed x (1, 0, 0) y (0, 1, 0) z (0, 0, 1) at (0, 0, 0)
component "04 Guition front glass — drawing reference" placed x (1, 0, 0) y (0, 1, 0) z (0, 0, 1) at (0, 0, 0)
component "05 Active 4.3 inch screen" placed x (1, 0, 0) y (0, 1, 0) z (0, 0, 1) at (0, 0, 0)
component "06 Guition PCB and connectors — illustrative detail" placed x (1, 0, 0) y (0, 1, 0) z (0, 0, 1) at (0, 0, 0)
component "M3 x 8 button screw — GEN-M3-BHCS-L8-AF2" placed x (1, 0, 0) y (0, 1, 0) z (0, 0, 1) at (6, 6, 56)
component "M3 insert OD4.2 x 5 — GEN-M3-HEATSET-OD4.2-L5" placed x (1, 0, 0) y (0, 1, 0) z (0, 0, 1) at (6, 6, 51.6)
component "Battery / FMA protected holder - owner-measured envelope" placed x (1, 0, 0) y (0, 1, 0) z (0, 0, 1) at (0, 0, 0)
component "Battery / 18650 cell A - owner-rated 3400 mAh" placed x (1, 0, 0) y (0, 1, 0) z (0, 0, 1) at (0, 0, 0)
component "Battery / 18650 cell B - owner-rated 3400 mAh" placed x (1, 0, 0) y (0, 1, 0) z (0, 0, 1) at (0, 0, 0)
component "Battery / red RCY disconnect body - provisional reference" placed x (1, 0, 0) y (0, 1, 0) z (0, 0, 1) at (0, 0, 0)
component "Battery / red RCY disconnect mate - provisional reference" placed x (1, 0, 0) y (0, 1, 0) z (0, 0, 1) at (0, 0, 0)
component "Carrier / removable electronics plate" placed x (1, 0, 0) y (0, 1, 0) z (0, 0, 1) at (0, 0, 0)
component "Carrier / future PCB allocation — layout pending" placed x (1, 0, 0) y (0, 1, 0) z (0, 0, 1) at (0, 0, 0)
component "M2 x 7 socket_cap screw — GEN-M2-SHCS-L7-AF1.5" placed x (1, 0, 0) y (0, 1, 0) z (0, 0, 1) at (6, 18, 47.25)
component "M2 insert OD3.2 x 4 — GEN-M2-HEATSET-OD3.2-L4" placed x (1, 0, 0) y (0, 1, 0) z (0, 0, 1) at (6, 18, 43.65)
component "Display / lower removable retainer concept" placed x (1, 0, 0) y (0, 1, 0) z (0, 0, 1) at (0, 0, 0)
component "Display / upper removable retainer concept" placed x (1, 0, 0) y (0, 1, 0) z (0, 0, 1) at (0, 0, 0)
component "M2 x 5 socket_cap screw — GEN-M2-SHCS-L5-AF1.5" placed x (1, 0, 0) y (0, 1, 0) z (0, 0, 1) at (52, 11, 22.3)
component "Controls / right 1NO power button body" placed x (1, 0, 0) y (0, 1, 0) z (0, 0, 1) at (0, 0, 0)
component "Controls / green momentary power cap" placed x (1, 0, 0) y (0, 1, 0) z (0, 0, 1) at (0, 0, 0)
component "M3 x 8 button screw — GEN-M3-BHCS-L8-AF2" placed x (1, 0, 0) y (0, 1, 0) z (0, 0, 1) at (69, 6, 56)
component "M3 x 8 button screw — GEN-M3-BHCS-L8-AF2" placed x (1, 0, 0) y (0, 1, 0) z (0, 0, 1) at (6, 119, 56)
component "M3 x 8 button screw — GEN-M3-BHCS-L8-AF2" placed x (1, 0, 0) y (0, 1, 0) z (0, 0, 1) at (69, 119, 56)
component "M3 insert OD4.2 x 5 — GEN-M3-HEATSET-OD4.2-L5" placed x (1, 0, 0) y (0, 1, 0) z (0, 0, 1) at (69, 6, 51.6)
component "M3 insert OD4.2 x 5 — GEN-M3-HEATSET-OD4.2-L5" placed x (1, 0, 0) y (0, 1, 0) z (0, 0, 1) at (6, 119, 51.6)
component "M3 insert OD4.2 x 5 — GEN-M3-HEATSET-OD4.2-L5" placed x (1, 0, 0) y (0, 1, 0) z (0, 0, 1) at (69, 119, 51.6)
component "M2 x 7 socket_cap screw — GEN-M2-SHCS-L7-AF1.5" placed x (1, 0, 0) y (0, 1, 0) z (0, 0, 1) at (6, 77, 47.25)
component "M2 x 7 socket_cap screw — GEN-M2-SHCS-L7-AF1.5" placed x (1, 0, 0) y (0, 1, 0) z (0, 0, 1) at (40, 14, 47.25)
component "M2 insert OD3.2 x 4 — GEN-M2-HEATSET-OD3.2-L4" placed x (1, 0, 0) y (0, 1, 0) z (0, 0, 1) at (6, 77, 43.65)
component "M2 insert OD3.2 x 4 — GEN-M2-HEATSET-OD3.2-L4" placed x (1, 0, 0) y (0, 1, 0) z (0, 0, 1) at (40, 14, 43.65)
component "M2 x 5 socket_cap screw — GEN-M2-SHCS-L5-AF1.5" placed x (1, 0, 0) y (0, 1, 0) z (0, 0, 1) at (14, 119, 22.3)
component "M2 insert OD3.2 x 4 — GEN-M2-HEATSET-OD3.2-L4" placed x (1, 0, 0) y (0, 1, 0) z (0, 0, 1) at (52, 11, 20.3)
component "M2 insert OD3.2 x 4 — GEN-M2-HEATSET-OD3.2-L4" placed x (1, 0, 0) y (0, 1, 0) z (0, 0, 1) at (14, 119, 20.3)
component "USB — removable metal faceplate — local 1.80 mm seat" placed x (1, 0, 0) y (0, 1, 0) z (0, 0, 1) at (0, 0, 0)
component "USB — removable panel insert and board supports" placed x (1, 0, 0) y (0, 1, 0) z (0, 0, 1) at (0, 0, 0)
component "USB — 0.60 mm daughterboard — layout provisional" placed x (1, 0, 0) y (0, 1, 0) z (0, 0, 1) at (0, 0, 0)
component "USB — GCT USB4720 metal shell — drawing reconstruction" placed x (1, 0, 0) y (0, 1, 0) z (0, 0, 1) at (0, 0, 0)
component "USB — GCT tongue and rear insulator — illustrative" placed x (1, 0, 0) y (0, 1, 0) z (0, 0, 1) at (0, 0, 0)
component "USB — GCT LIM gasket — drawing reference" placed x (1, 0, 0) y (0, 1, 0) z (0, 0, 1) at (0, 0, 0)
component "USB — contact detail — illustrative only" placed x (1, 0, 0) y (0, 1, 0) z (0, 0, 1) at (0, 0, 0)
component "M2 x 4 socket_cap screw — GEN-M2-SHCS-L4-AF1.5" placed x (1, 0, 0) y (0, 1, 0) z (0, 0, 1) at (63.7, 10.4, 27.3)
component "M2 x 6 socket_cap screw — GEN-M2-SHCS-L6-AF1.5" placed x (0, 0, -1) y (0, 1, 0) z (1, 0, 0) at (74.9, 8.25, 21.25)
component "USB — removable rear housing clamp" placed x (1, 0, 0) y (0, 1, 0) z (0, 0, 1) at (0, 0, 0)
component "Chamber / removable internal lid" placed x (1, 0, 0) y (0, 1, 0) z (0, 0, 1) at (0, 0, 0)
component "Sensor / AO2 sideways body and neck" placed x (1, 0, 0) y (0, 1, 0) z (0, 0, 1) at (0, 0, 0)
component "Sensor / AO2 connector allowance" placed x (1, 0, 0) y (0, 1, 0) z (0, 0, 1) at (0, 0, 0)
component "Sensor / ZE07-CO rotated total envelope" placed x (1, 0, 0) y (0, 1, 0) z (0, 0, 1) at (0, 0, 0)
component "Sensor / MD62 rotated body envelope" placed x (1, 0, 0) y (0, 1, 0) z (0, 0, 1) at (0, 0, 0)
component "Sensor / MD62 27 mm lead allowance" placed x (1, 0, 0) y (0, 1, 0) z (0, 0, 1) at (0, 0, 0)
component "Sensor / GYBMEP wired module envelope" placed x (1, 0, 0) y (0, 1, 0) z (0, 0, 1) at (0, 0, 0)
component "Gas / left inlet fitting reference" placed x (1, 0, 0) y (0, 1, 0) z (0, 0, 1) at (0, 0, 0)
component "Gas / right exhaust fitting reference" placed x (1, 0, 0) y (0, 1, 0) z (0, 0, 1) at (0, 0, 0)
component "Chamber / sealed wire feedthrough concept" placed x (1, 0, 0) y (0, 1, 0) z (0, 0, 1) at (0, 0, 0)
component "M2 x 4 socket_cap screw — GEN-M2-SHCS-L4-AF1.5" placed x (1, 0, 0) y (0, 1, 0) z (0, 0, 1) at (59.5, 21.6, 27.3)
component "M2 insert OD3.2 x 4 — GEN-M2-HEATSET-OD3.2-L4" placed x (1, 0, 0) y (0, 1, 0) z (0, 0, 1) at (63.7, 10.4, 26.7)
component "M2 insert OD3.2 x 4 — GEN-M2-HEATSET-OD3.2-L4" placed x (1, 0, 0) y (0, 1, 0) z (0, 0, 1) at (59.5, 21.6, 26.7)
component "M2 x 6 socket_cap screw — GEN-M2-SHCS-L6-AF1.5" placed x (0, 0, -1) y (0, 1, 0) z (1, 0, 0) at (74.9, 23.75, 30.95)
component "M2 insert OD3.2 x 4 — GEN-M2-HEATSET-OD3.2-L4" placed x (0, 0, -1) y (0, 1, 0) z (1, 0, 0) at (72.6, 8.25, 21.25)
component "M2 insert OD3.2 x 4 — GEN-M2-HEATSET-OD3.2-L4" placed x (0, 0, -1) y (0, 1, 0) z (1, 0, 0) at (72.6, 23.75, 30.95)
component "M2 insert OD3.2 x 4 — GEN-M2-HEATSET-OD3.2-L4" placed x (1, 0, 0) y (0, 1, 0) z (0, 0, 1) at (69.3, 16, 43.2)
component "M2 x 5 socket_cap screw — GEN-M2-SHCS-L5-AF1.5" placed x (1, 0, 0) y (0, 1, 0) z (0, 0, 1) at (17.4, 92.6, 50.8)
component "M2 x 5 socket_cap screw — GEN-M2-SHCS-L5-AF1.5" placed x (1, 0, 0) y (0, 1, 0) z (0, 0, 1) at (12.9, 110.6, 50.8)
component "M2 x 5 socket_cap screw — GEN-M2-SHCS-L5-AF1.5" placed x (1, 0, 0) y (0, 1, 0) z (0, 0, 1) at (66.5, 83.5, 50.8)
component "M2 x 5 socket_cap screw — GEN-M2-SHCS-L5-AF1.5" placed x (1, 0, 0) y (0, 1, 0) z (0, 0, 1) at (66.5, 110.5, 50.8)
component "M2 x 5 socket_cap screw — GEN-M2-SHCS-L5-AF1.5" placed x (1, 0, 0) y (0, 1, 0) z (0, 0, 1) at (51.2, 34, 50.8)
component "M2 x 5 socket_cap screw — GEN-M2-SHCS-L5-AF1.5" placed x (1, 0, 0) y (0, 1, 0) z (0, 0, 1) at (66.5, 34, 50.8)
component "M2 insert OD3.2 x 4 — GEN-M2-HEATSET-OD3.2-L4" placed x (1, 0, 0) y (0, 1, 0) z (0, 0, 1) at (17.4, 92.6, 48.8)
component "M2 insert OD3.2 x 4 — GEN-M2-HEATSET-OD3.2-L4" placed x (1, 0, 0) y (0, 1, 0) z (0, 0, 1) at (12.9, 110.6, 48.8)
component "M2 insert OD3.2 x 4 — GEN-M2-HEATSET-OD3.2-L4" placed x (1, 0, 0) y (0, 1, 0) z (0, 0, 1) at (66.5, 83.5, 48.8)
component "M2 insert OD3.2 x 4 — GEN-M2-HEATSET-OD3.2-L4" placed x (1, 0, 0) y (0, 1, 0) z (0, 0, 1) at (66.5, 110.5, 48.8)
component "M2 insert OD3.2 x 4 — GEN-M2-HEATSET-OD3.2-L4" placed x (1, 0, 0) y (0, 1, 0) z (0, 0, 1) at (51.2, 34, 48.8)
component "M2 insert OD3.2 x 4 — GEN-M2-HEATSET-OD3.2-L4" placed x (1, 0, 0) y (0, 1, 0) z (0, 0, 1) at (66.5, 34, 48.8)
component "M2 x 5 socket_cap screw — GEN-M2-SHCS-L5-AF1.5" placed x (1, 0, 0) y (0, 1, 0) z (0, 0, 1) at (8.8, 94.7, 48.8)
component "M2 x 5 socket_cap screw — GEN-M2-SHCS-L5-AF1.5" placed x (1, 0, 0) y (0, 1, 0) z (0, 0, 1) at (59.2, 115.4, 48.8)
component "M2 insert OD3.2 x 4 — GEN-M2-HEATSET-OD3.2-L4" placed x (1, 0, 0) y (0, 1, 0) z (0, 0, 1) at (8.8, 94.7, 46.8)
component "M2 insert OD3.2 x 4 — GEN-M2-HEATSET-OD3.2-L4" placed x (1, 0, 0) y (0, 1, 0) z (0, 0, 1) at (59.2, 115.4, 46.8)
component "Chamber / sealed L cartridge concept" placed x (1, 0, 0) y (0, 1, 0) z (0, 0, 1) at (0, 0, 0)
component "M2 x 5 socket_cap screw — GEN-M2-SHCS-L5-AF1.5" placed x (1, 0, 0) y (0, 1, 0) z (0, 0, 1) at (69.3, 16, 45.2)
equation "CaseWidth = 75 mm" comment "Initial compact housing width"
equation "CaseHeight = 125 mm" comment "Initial compact housing height"
equation "CaseDepth = 56 mm" comment "Housing including one rear cover"
equation "Wall = 2.4 mm" comment "Nominal printed shell wall; minimum check >=2 mm"
equation "RearInset = 0.25 mm" comment "Gentle inward taper per outer edge"
equation "CornerRadius = 6 mm" comment "Soft longitudinal corner radius"
equation "Cover = 2.4 mm" comment "Single rear cover thickness"
equation "CoverGap = 0.2 mm" comment "Provisional seating gap; not a weather seal"
equation "DisplayWidth = 69.3 mm" comment "Owner measured; remaining factory casing retained"
equation "DisplayHeight = 116.8 mm" comment "Owner measured"
equation "DisplayDepth = 13.7 mm" comment "Owner measured with only factory rear panel removed"
equation "DisplayX = ( CaseWidth - DisplayWidth ) / 2" comment "Centred factory display"
equation "DisplayY = ( CaseHeight - DisplayHeight ) / 2" comment "Centred factory display"
equation "DisplayFront = 0.4 mm" comment "Slightly recessed from printed front rim"
equation "DisplayFit = 0.4 mm" comment "Provisional clearance per side of front removable display"
equation "GlassWidth = 66.8 mm" comment "Published glass reference; physical confirmation pending"
equation "GlassHeight = 114.4 mm" comment "Published glass reference"
equation "ActiveWidth = 56.16 mm" comment "Published active screen width"
equation "ActiveHeight = 93.60 mm" comment "Published active screen height"
equation "HolderWidth = 42 mm" comment "Owner measured occupied FMA holder"
equation "HolderHeight = 80.4 mm" comment "Owner measured occupied FMA holder"
equation "HolderDepth = 20.35 mm" comment "Owner measured maximum occupied thickness"
equation "HolderX = 3 mm" comment "Battery is behind lower right portion of screen"
equation "HolderY = 4.2 mm" comment "Occupied battery lower edge"
equation "HolderZ = 16.7 mm" comment "Display and battery clearance"
equation "ChamberWall = 2 mm" comment "Concept chamber wall; seal qualification pending"
equation "ChamberFront = 16.5 mm" comment "Front of independent rear sampling cartridge"